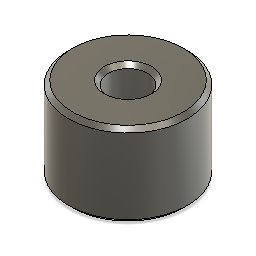
Enderson (Autodesk Fusion 360 archive; units mm, degrees)
design "Carriage Spacer 10.5mm"
Autodesk Fusion 360 part; units mm, degrees
sketch "Sketch1" plane through (0, 0, 0) normal (0, 1, 0) x (1, 0, 0)
  circle A0 centre (0, 0) radius 7.5
  circle A1 centre (0, 0) radius 2.5
  dimension "d1" = 15
  dimension "d2" = 5
  constraint coincident A0.centre A1.centre
  measures "d1" diameter of A0
  measures "d2" diameter of A1
extrude "Extrude1" add sketch "Sketch1" against normal blind 10.5
chamfer "Chamfer1" distance 0.5 angle 45 2 edges at (-6.9925, 0, 2.7121) (-6.9925, -10.5, -2.7121)
chamfer "Chamfer2" distance 0.5 angle 45 2 edges at (-2.3308, -10.5, 0.904) (-2.3308, 0, -0.904)

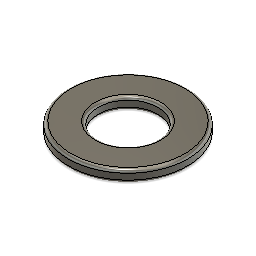
design "M5 Washer 5mm x 10mm x 1mm"
Autodesk Fusion 360 part; units mm, degrees
sketch "Sketch1" plane through (0, 0, 0) normal (0, 1, 0) x (1, 0, 0)
  circle A0 centre (0, 0) radius 2.5
  circle A1 centre (0, 0) radius 5
  dimension "d1" = 5
  dimension "d2" = 10
  constraint coincident A0.centre A1.centre
  constraint concentric A0 A1
  measures "d1" diameter of A0
  measures "d2" diameter of A1
extrude "Extrude1" add sketch "Sketch1" along normal blind 1
fillet "Fillet1" radius 0.25 4 edges at (-4.6616, 1, 1.8081) (-4.6616, 0, 1.8081) (-2.3308, 1, -0.904) (-2.3308, 0, -0.904)

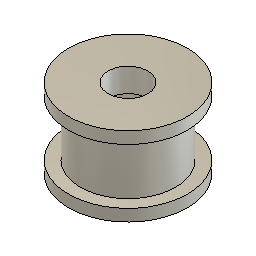
design "Gates GT2 Toothed Idler 6mm"
Autodesk Fusion 360 part; units mm, degrees
sketch "Sketch1" plane through (0, 0, 0) normal (0, 0, 1) x (1, 0, 0)
  line L0 (-6, 8.5) -> (6, 8.5)
  line L1 (6, 8.5) -> (6, 1.5)
  line L2 (6, 1.5) -> (-6, 1.5)
  line L3 (-6, 1.5) -> (-6, 8.5)
  line L4 (-7.5, 10) -> (7.5, 10)
  line L5 (7.5, 10) -> (7.5, 8.5)
  line L6 (7.5, 8.5) -> (-7.5, 8.5)
  line L7 (-7.5, 8.5) -> (-7.5, 10)
  line L8 (-7.5, 1.5) -> (7.5, 1.5)
  line L9 (7.5, 1.5) -> (7.5, 0)
  line L10 (7.5, 0) -> (-7.5, 0)
  line L11 (-7.5, 0) -> (-7.5, 1.5)
  line L12 (0, 0) -> (0, 10)
  line L13 (2.5, 10) -> (4.5, 10)
  line L14 (4.5, 10) -> (4.5, 7)
  line L15 (4.5, 7) -> (2.5, 7)
  line L16 (2.5, 7) -> (2.5, 10)
  line L17 (0, 5) -> (6, 5) construction
  line L18 (2.5, 0) -> (4.5, 0)
  line L19 (4.5, 0) -> (4.5, 3)
  line L20 (4.5, 3) -> (2.5, 3)
  line L21 (2.5, 3) -> (2.5, 0)
  line L22 (-2.5, 7) -> (-2.5, 10)
  line L23 (-2.5, 10) -> (-4.5, 10)
  line L24 (-4.5, 10) -> (-4.5, 7)
  line L25 (-4.5, 7) -> (-2.5, 7)
  line L26 (-2.5, 3) -> (-2.5, 0)
  line L27 (-2.5, 0) -> (-4.5, 0)
  line L28 (-4.5, 3) -> (-2.5, 3)
  line L29 (-4.5, 0) -> (-4.5, 3)
  line L30 (3.5, 7) -> (3.5, 3)
  line L31 (-3.5, 7) -> (-3.5, 3)
  dimension "d1" = 15
  dimension "d2" = 1.5
  dimension "d3" = 1.5
  dimension "d4" = 12
  dimension "d5" = 7
  dimension "d6" = 5
  dimension "d7" = 9
  dimension "d8" = 3
  dimension "d9" = 7
  constraint horizontal L0
  constraint vertical L1
  constraint horizontal L2
  constraint vertical L3
  constraint horizontal L4
  constraint vertical L5
  constraint horizontal L6
  constraint vertical L7
  constraint horizontal L8
  constraint vertical L9
  constraint horizontal L10
  constraint vertical L11
  constraint coincident L12.start origin
  constraint perpendicular L0 L12
  constraint midpoint L12.start L10
  constraint midpoint L2 L8
  constraint midpoint L0 L6
  constraint midpoint L4 L12.end
  constraint collinear L5 L9
  constraint horizontal L13
  constraint vertical L14
  constraint horizontal L15
  constraint vertical L16
  constraint midpoint L12 L17.start
  constraint midpoint L1 L17.end
  constraint symmetric L13.start L17 L18.start
  constraint symmetric L13.end L17 L18.end
  constraint symmetric L14.end L17 L19.end
  constraint symmetric L15.end L17 L20.end
  constraint coincident L4 L13.start
  constraint symmetric L12 L13.start L22.end
  constraint symmetric L12 L13.end L23.end
  constraint symmetric L12 L14.end L24.end
  constraint symmetric L12 L15.end L22.start
  constraint symmetric L12 L18.start L26.end
  constraint symmetric L12 L18.end L27.end
  constraint symmetric L12 L19.end L28.start
  constraint symmetric L12 L20.end L26.start
  constraint coincident L15 L30.start
  constraint coincident L20 L30.end
  constraint perpendicular L20 L30
  constraint symmetric L12 L30.start L31.start
  constraint symmetric L12 L30.end L31.end
  measures "d1" distance of L5.end L6.end
  measures "d2" distance of L0 L4
  measures "d3" distance of L2 L10
  measures "d4" distance of L1 L3
  measures "d5" distance of L6 L8
  measures "d6" distance of L16 L22
  measures "d7" distance of L14 L24
  measures "d8" distance of L4 L15
  measures "d9" distance of L30 L31
revolve "Revolve1" add sketch "Sketch1" angle 360 about axis through (0, 0, 0) along (0, 1, 0) contours L0 L4 L6 L13 L14 L16 | L0 L6 L14 L15 L16 | L0 L4 L5 L6 L14 | L0 L1 L2 L6 L8 L14 L15 L19 L20 L30 | L2 L8 L19 L20 L21 | L2 L8 L10 L18 L19 L21 | L2 L8 L9 L10 L19
equation "d3 = d2"

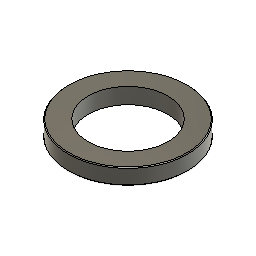
design "Nylon Washer"
Autodesk Fusion 360 part; units mm, degrees
sketch "Sketch1" plane through (0, 0, 0) normal (0, 1, 0) x (1, 0, 0)
  circle A0 centre (0, 0) radius 3.75
  circle A1 centre (0, 0) radius 2.5
  dimension "d1" = 7.5
  dimension "d2" = 5
  constraint coincident A0.centre A1.centre
  constraint concentric A0 A1
  measures "d1" diameter of A0
  measures "d2" diameter of A1
extrude "Extrude1" add sketch "Sketch1" along normal blind 1
chamfer "Chamfer1" distance 0.05 angle 45 2 edges at (-3.4962, 1, 1.3561) (-3.4962, 0, 1.3561)
